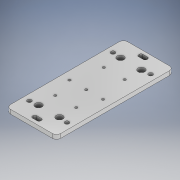
# Autodesk Inventor part: Y-Axis_back_plate_top
Saved by Autodesk Inventor 2021.3 (Build 253353000, 353)
## iProperties
Created: 2021-04-15
Part Number: Y-Axis_back_plate_top
Material: PET Plastic
Document SubType Name: Modeling
Designer: Fabijan_Sven
Density: 1.541 g/cm^3
Appearance: Aluminum - Polished
Mass: 61.3035 g
Surface Area: 192.821 cm^2
Volume: 39.7816 cm^3
Author: Fabijan_Sven
Autodesk Inventor part; units mm, degrees
ref_plane "YZ Plane" through (0, 0, 0) normal (1, 0, 0) x (0, 1, 0)
ref_plane "XZ Plane" through (0, 0, 0) normal (0, 1, 0) x (-1, 0, 0)
ref_plane "XY Plane" through (0, 0, 0) normal (0, 0, 1) x (1, 0, 0)
sketch "Sketch1" plane through (0, 0, 0) normal (0, 1, 0) x (-1, 0, 0)
  line L0 (0, 0) -> (60, 0)
  line L1 (60, 0) -> (60, -140)
  line L2 (60, -140) -> (0, -140)
  line L3 (0, -140) -> (0, 0)
  line L4 (30, -20.8594) -> (30, -183.1932) construction
  line L5 (42.5, -21.7206) -> (42.5, -191.0157) construction
  line L6 (17.5, -21.7206) -> (17.5, -184.1979) construction
  circle A0 centre (42.5, -21) radius 4
  circle A1 centre (42.5, -41) radius 1.5
  circle A2 centre (42.5, -99) radius 1.5
  circle A3 centre (42.5, -119) radius 4
  circle A4 centre (17.5, -99) radius 1.5
  circle A5 centre (17.5, -119) radius 4
  circle A6 centre (17.5, -41) radius 1.5
  circle A7 centre (17.5, -21) radius 4
  dimension "d0" = 140
  dimension "d1" = 60
  dimension "d2" = 30
  dimension "d3" = 12.5
  dimension "d4" = 12.5
  dimension "d5" = 8
  dimension "d6" = 3
  dimension "d7" = 3
  dimension "d8" = 8
  dimension "d9" = 3
  dimension "d10" = 8
  dimension "d11" = 3
  dimension "d12" = 8
  dimension "d13" = 20
  dimension "d14" = 20
  dimension "d15" = 20
  dimension "d16" = 20
  dimension "d17" = 21
  dimension "d18" = 21
  dimension "d19" = 21
  dimension "d20" = 21
  constraints: 14 end point, 8 centre point, 8 point on line, 3 vertical, 2 parallel, 1 horizontal, 1 perpendicular
  measures "d0" distance of L0.end L1.end
  measures "d1" distance of L1.end L2.end
  measures "d2" distance between parallel lines of L4 L1
  measures "d3" distance between parallel lines of L5 L4
  measures "d4" distance between parallel lines of L6 L4
  measures "d5" diameter of A0
  measures "d6" diameter of A1
  measures "d7" diameter of A2
  measures "d8" diameter of A3
  measures "d9" diameter of A4
  measures "d10" diameter of A5
  measures "d11" diameter of A6
  measures "d12" diameter of A7
  measures "d13" distance of A1.centre A0.centre
  measures "d14" distance of A6.centre A7.centre
  measures "d15" distance of A3.centre A2.centre
  measures "d16" distance of A5.centre A4.centre
  measures "d17" distance from line of L0 A0.centre
  measures "d18" distance from line of L0 A7.centre
  measures "d19" distance from line of L2 A3.centre
  measures "d20" distance from line of A5.centre L2
extrude "Extrusion1" add sketch "Sketch1" along normal blind 5
sketch "Sketch2" plane through (0, 0, 0) normal (0, -1, 0) x (1, 0, 0)
  circle A0 centre (-52.5, -120) radius 2.5
  circle A1 centre (-52.5, -20) radius 2.5
  circle A2 centre (-7.5, -120) radius 2.5
  circle A3 centre (-7.5, -20) radius 2.5
  line L0 (-60, -140) -> (-60, 0) projected
  line L1 (0, -140) -> (-60, -140) projected
  line L2 (-60, 0) -> (0, 0) projected
  line L3 (0, 0) -> (0, -140) projected
  dimension "d23" = 5
  dimension "d24" = 5
  dimension "d25" = 5
  dimension "d26" = 5
  dimension "d27" = 7.5
  dimension "d28" = 20
  dimension "d29" = 7.5
  dimension "d30" = 20
  dimension "d31" = 20
  dimension "d32" = 7.5
  dimension "d33" = 20
  dimension "d34" = 7.5
  constraints: 4 centre point
  measures "d23" diameter of A0
  measures "d24" diameter of A1
  measures "d25" diameter of A2
  measures "d26" diameter of A3
  measures "d27" distance from line of L0 A0.centre
  measures "d28" distance from line of L1 A0.centre
  measures "d29" distance from line of L0 A1.centre
  measures "d30" distance from line of L2 A1.centre
  measures "d31" distance from line of L2 A3.centre
  measures "d32" distance from line of L3 A3.centre
  measures "d33" distance from line of L1 A2.centre
  measures "d34" distance from line of L3 A2.centre
extrude "Extrusion2" cut sketch "Sketch2" against normal blind 10 contours A0 | A1 | A2 | A3
sketch "Sketch3" plane through (0, 0, 0) normal (0, -1, 0) x (1, 0, 0)
  line L0 (-68.3542, -70) -> (15.9682, -70) construction
  line L1 (0, -140) -> (-60, -140) projected
  line L2 (-35, -136) -> (-25, -136)
  line L3 (-25, -136) -> (-25, -131)
  line L4 (-25, -131) -> (-35, -131)
  line L5 (-35, -131) -> (-35, -136)
  line L6 (-60, -140) -> (-60, 0) projected
  line L7 (-35, -4) -> (-25, -4)
  line L8 (-25, -4) -> (-25, -9)
  line L9 (-25, -9) -> (-35, -9)
  line L10 (-35, -9) -> (-35, -4)
  point P0 (0, 0)
  dimension "d40" = 70
  dimension "d41" = 10
  dimension "d42" = 25
  dimension "d43" = 4
  dimension "d44" = 5
  constraints: 18 end point, 4 symmetric about line, 2 horizontal, 2 parallel, 1 perpendicular
  measures "d40" distance between parallel lines of L1 L0
  measures "d41" distance of L2.start L2.end
  measures "d42" distance between parallel lines of L6 L5
  measures "d43" distance between parallel lines of L1 L2
  measures "d44" distance between parallel lines of L2 L4
extrude "Extrusion3" cut sketch "Sketch3" against normal blind 10
fillet "Fillet2" radius 5 4 edges at (0, 2.5, -140) (-60, 2.5, -140) (-60, 2.5, 0) (0, 2.5, 0)
sketch "Sketch4" plane through (0, 5, 0) normal (0, 1, 0) x (1, 0, 0)
  circle A0 centre (-10, 65.5) radius 1.5
  circle A1 centre (-30, 65.5) radius 1.5
  circle A2 centre (-50, 65.5) radius 1.5
  line L0 (3.8133, 65.5) -> (-51.9818, 65.5) construction
  line L1 (-55, 0) -> (-5, 0) projected
  line L2 (0, 5) -> (0, 135) projected
  point P0 (0, 0)
  dimension "d49" = 3
  dimension "d50" = 3
  dimension "d51" = 3
  dimension "d52" = 65.5
  dimension "d53" = 10
  dimension "d54" = 30
  dimension "d55" = 50
  constraints: 3 centre point, 3 point on line, 2 end point, 1 horizontal
  measures "d49" diameter of A0
  measures "d50" diameter of A1
  measures "d51" diameter of A2
  measures "d52" distance between parallel lines of L0 L1
  measures "d53" distance from line of A0.centre L2
  measures "d54" distance from line of A1.centre L2
  measures "d55" distance from line of L2 A2.centre
extrude "Extrusion4" cut sketch "Sketch4" against normal blind 10
fillet "Fillet3" radius 2 8 edges at (-25, 2.5, -131) (-25, 2.5, -136) (-35, 2.5, -136) (-35, 2.5, -131) (-25, 2.5, -9) (-25, 2.5, -4) (-35, 2.5, -4) (-35, 2.5, -9)
equation "\"d2\" = 0.5 * d1"
equation "\"d4\" = d3"
equation "\"d8\" = d5"
equation "\"d10\" = d5"
equation "\"d12\" = d5"
equation "\"d14\" = d13"
equation "\"d15\" = d13"
equation "\"d16\" = d13"
equation "\"d18\" = d17"
equation "\"d19\" = d17"
equation "\"d20\" = d17"
equation "\"d29\" = d27"
equation "\"d30\" = d28"
equation "\"d31\" = d28"
equation "\"d32\" = d27"
equation "\"d33\" = d28"
equation "\"d34\" = d27"
body "Solid1"
